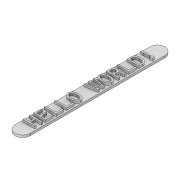
# Autodesk Inventor part: hello_world
Saved by Autodesk Inventor 2021 (Build 250183000, 183)
## iProperties
Created: 2021-09-21
Part Number: hello_world
Material: Generic
Document SubType Name: Modeling
Designer: Administrator
Density: 1 g/cm^3
Appearance: Default
Author: Administrator
Autodesk Inventor part; units mm, degrees
ref_plane "YZ Plane" through (0, 0, 0) normal (1, 0, 0) x (0, 1, 0)
ref_plane "XZ Plane" through (0, 0, 0) normal (0, 1, 0) x (-1, 0, 0)
ref_plane "XY Plane" through (0, 0, 0) normal (0, 0, 1) x (1, 0, 0)
sketch "Sketch1" plane through (0, 0, 0) normal (0, 1, 0) x (-1, 0, 0)
  line L0 (25, -250) -> (-25, -250)
  line L1 (-25, -250) -> (-25, 250)
  line L2 (-25, 250) -> (25, 250)
  line L3 (25, 250) -> (25, -250)
  line L4 (25, -250) -> (-25, 250) construction
  line L5 (-25, -250) -> (25, 250) construction
  point P0 (0, 0)
  dimension "d0" = 50
  dimension "d1" = 500
  constraints: 12 end point, 2 midpoint, 2 parallel, 1 horizontal, 1 perpendicular
  measures "d0" distance of L1.end L2.end
  measures "d1" distance of L0.end L1.end
extrude "Extrusion1" add sketch "Sketch1" along normal blind 7.5
fillet "Fillet1" radius 25 4 edges at (25, 3.75, 250) (-25, 3.75, 250) (25, 3.75, -250) (-25, 3.75, -250)
sketch "Sketch2" plane through (0, 7.5, 0) normal (0, 1, 0) x (1, 0, 0)
  line L0 (-21.1138, -208.405) -> (-21.1138, 208.4051) construction
  line L1 (-21.1138, 208.4051) -> (21.114, 208.4051) construction
  line L2 (21.114, 208.4051) -> (21.114, -208.405) construction
  line L3 (21.114, -208.405) -> (-21.1138, -208.405) construction
  line L4 (-25, 225) -> (-25, -225) projected
  arc A0 (-25, -225) -> (25, -225) centre (0, -225) ccw projected
  arc A1 (25, 225) -> (-25, 225) centre (0, 225) ccw projected
  line L5 (20.0001, -204.4219) -> (-19.9999, -204.4219)
  line L6 (-19.9999, -204.4219) -> (-19.9999, -199.0548)
  line L7 (-19.9999, -199.0548) -> (-3.6961, -199.0548)
  line L8 (-3.6961, -199.0548) -> (-3.6961, -183.0548)
  line L9 (-3.6961, -183.0548) -> (-19.9999, -183.0548)
  line L10 (-19.9999, -183.0548) -> (-19.9999, -177.7215)
  line L11 (-19.9999, -177.7215) -> (20.0001, -177.7215)
  line L12 (20.0001, -177.7215) -> (20.0001, -183.0548)
  line L13 (20.0001, -183.0548) -> (1.1984, -183.0548)
  line L14 (1.1984, -183.0548) -> (1.1984, -199.0548)
  line L15 (1.1984, -199.0548) -> (20.0001, -199.0548)
  line L16 (20.0001, -199.0548) -> (20.0001, -204.4219)
  line L17 (20.0001, -168.4388) -> (-19.9999, -168.4388)
  line L18 (-19.9999, -168.4388) -> (-19.9999, -143.5274)
  line L19 (-19.9999, -143.5274) -> (-15.1729, -143.5274)
  line L20 (-15.1729, -143.5274) -> (-15.1729, -163.1054)
  line L21 (-15.1729, -163.1054) -> (-3.156, -163.1054)
  line L22 (-3.156, -163.1054) -> (-3.156, -145.2489)
  line L23 (-3.156, -145.2489) -> (1.6372, -145.2489)
  line L24 (1.6372, -145.2489) -> (1.6372, -163.1054)
  line L25 (1.6372, -163.1054) -> (15.1731, -163.1054)
  line L26 (15.1731, -163.1054) -> (15.1731, -143.0885)
  line L27 (15.1731, -143.0885) -> (20.0001, -143.0885)
  line L28 (20.0001, -143.0885) -> (20.0001, -168.4388)
  line L29 (20.0001, -133.2658) -> (-19.9999, -133.2658)
  line L30 (-19.9999, -133.2658) -> (-19.9999, -127.9662)
  line L31 (-19.9999, -127.9662) -> (15.1731, -127.9662)
  line L32 (15.1731, -127.9662) -> (15.1731, -107.578)
  line L33 (15.1731, -107.578) -> (20.0001, -107.578)
  line L34 (20.0001, -107.578) -> (20.0001, -133.2658)
  line L35 (20.0001, -98.5316) -> (-19.9999, -98.5316)
  line L36 (-19.9999, -98.5316) -> (-19.9999, -93.232)
  line L37 (-19.9999, -93.232) -> (15.1731, -93.232)
  line L38 (15.1731, -93.232) -> (15.1731, -72.8438)
  line L39 (15.1731, -72.8438) -> (20.0001, -72.8438)
  line L40 (20.0001, -72.8438) -> (20.0001, -98.5316)
  spline S0 degree 2 poles (-0.0168, -66.9366) (-9.9746, -66.9366) (-21.1138, -59.0717) (-21.1138, -52.1181) knots 0 0 0 1 2 2 2
  spline S1 degree 2 poles (-21.1138, -52.1181) (-21.1138, -45.1982) (-9.8733, -37.2995) (-0.0168, -37.2995) knots 0 0 0 1 2 2 2
  spline S2 degree 2 poles (-0.0168, -37.2995) (9.8735, -37.2995) (21.114, -45.1982) (21.114, -52.1181) knots 0 0 0 1 2 2 2
  spline S3 degree 2 poles (21.114, -52.1181) (21.114, -59.0379) (9.8735, -66.9366) (-0.0168, -66.9366) knots 0 0 0 1 2 2 2
  spline S4 degree 2 poles (-0.0168, -61.4008) (7.6119, -61.4008) (16.287, -56.405) (16.287, -52.1181) knots 0 0 0 1 2 2 2
  spline S5 degree 2 poles (16.287, -52.1181) (16.287, -47.8312) (7.5781, -42.8354) (-0.0168, -42.8354) knots 0 0 0 1 2 2 2
  spline S6 degree 2 poles (-0.0168, -42.8354) (-7.6117, -42.8354) (-16.3206, -47.8312) (-16.3206, -52.1181) knots 0 0 0 1 2 2 2
  spline S7 degree 2 poles (-16.3206, -52.1181) (-16.3206, -56.405) (-7.6455, -61.4008) (-0.0168, -61.4008) knots 0 0 0 1 2 2 2
  line L41 (20.0001, 6.4473) -> (-20.0674, -0.4388)
  line L42 (-20.0674, -0.4388) -> (-20.0674, 4.287)
  line L43 (-20.0674, 4.287) -> (13.9916, 9.249)
  line L44 (13.9916, 9.249) -> (-20.0674, 14.7849)
  line L45 (-20.0674, 14.7849) -> (-20.0674, 19.8144)
  line L46 (-20.0674, 19.8144) -> (13.9916, 25.5191)
  line L47 (13.9916, 25.5191) -> (-20.0674, 30.4811)
  line L48 (-20.0674, 30.4811) -> (-20.0674, 35.1055)
  line L49 (-20.0674, 35.1055) -> (20.0001, 28.0507)
  line L50 (20.0001, 28.0507) -> (20.0001, 23.2237)
  line L51 (20.0001, 23.2237) -> (-14.7341, 17.249)
  line L52 (-14.7341, 17.249) -> (20.0001, 11.5444)
  line L53 (20.0001, 11.5444) -> (20.0001, 6.4473)
  spline S8 degree 2 poles (-0.0168, 37.2659) (-9.9746, 37.2659) (-21.1138, 45.1309) (-21.1138, 52.0845) knots 0 0 0 1 2 2 2
  spline S9 degree 2 poles (-21.1138, 52.0845) (-21.1138, 59.0043) (-9.8733, 66.903) (-0.0168, 66.903) knots 0 0 0 1 2 2 2
  spline S10 degree 2 poles (-0.0168, 66.903) (9.8735, 66.903) (21.114, 59.0043) (21.114, 52.0845) knots 0 0 0 1 2 2 2
  spline S11 degree 2 poles (21.114, 52.0845) (21.114, 45.1646) (9.8735, 37.2659) (-0.0168, 37.2659) knots 0 0 0 1 2 2 2
  spline S12 degree 2 poles (-0.0168, 42.8018) (7.6119, 42.8018) (16.287, 47.7975) (16.287, 52.0845) knots 0 0 0 1 2 2 2
  spline S13 degree 2 poles (16.287, 52.0845) (16.287, 56.3714) (7.5781, 61.3672) (-0.0168, 61.3672) knots 0 0 0 1 2 2 2
  spline S14 degree 2 poles (-0.0168, 61.3672) (-7.6117, 61.3672) (-16.3206, 56.3714) (-16.3206, 52.0845) knots 0 0 0 1 2 2 2
  spline S15 degree 2 poles (-16.3206, 52.0845) (-16.3206, 47.7975) (-7.6455, 42.8018) (-0.0168, 42.8018) knots 0 0 0 1 2 2 2
  line L54 (20.0001, 73.9579) -> (-19.9999, 73.9579)
  line L55 (-19.9999, 73.9579) -> (-19.9999, 87.325)
  spline S16 degree 2 poles (-19.9999, 87.325) (-19.9999, 93.2321) (-14.1603, 99.4431) (-8.5906, 99.4431) knots 0 0 0 1 2 2 2
  spline S17 degree 2 poles (-8.5906, 99.4431) (-5.2826, 99.4431) (-0.7257, 96.7764) (0.4895, 94.1773) knots 0 0 0 1 2 2 2
  spline S18 degree 2 poles (0.4895, 94.1773) (1.1646, 96.3376) (4.1013, 98.2617) (7.8144, 98.5317) knots 0 0 0 1 2 2 2
  line L56 (7.8144, 98.5317) -> (14.3292, 98.9368)
  spline S19 degree 2 poles (14.3292, 98.9368) (16.422, 99.0718) (18.3798, 99.8819) (18.8862, 100.7258) knots 0 0 0 1 2 2 2
  line L57 (18.8862, 100.7258) -> (20.0001, 100.7258)
  line L58 (20.0001, 100.7258) -> (20.0001, 94.6499)
  spline S20 degree 2 poles (20.0001, 94.6499) (19.3587, 94.2785) (16.7596, 93.7722) (14.5655, 93.6372) knots 0 0 0 1 2 2 2
  line L59 (14.5655, 93.6372) -> (9.4009, 93.3334)
  spline S21 degree 2 poles (9.4009, 93.3334) (5.4853, 93.1309) (3.1224, 90.3629) (3.1224, 84.7933) knots 0 0 0 1 2 2 2
  line L60 (3.1224, 84.7933) -> (3.1224, 79.2912)
  line L61 (3.1224, 79.2912) -> (20.0001, 79.2912)
  line L62 (20.0001, 79.2912) -> (20.0001, 73.9579)
  line L63 (-15.1054, 85.8397) -> (-15.1054, 79.2912)
  line L64 (-15.1054, 79.2912) -> (-1.7721, 79.2912)
  line L65 (-1.7721, 79.2912) -> (-1.7721, 85.4684)
  spline S22 degree 2 poles (-1.7721, 85.4684) (-1.7721, 90.1942) (-4.8776, 93.9072) (-8.4894, 93.9072) knots 0 0 0 1 2 2 2
  spline S23 degree 2 poles (-8.4894, 93.9072) (-12.0337, 93.9072) (-15.1054, 90.2279) (-15.1054, 85.8397) knots 0 0 0 1 2 2 2
  line L66 (20.0001, 109.8735) -> (-19.9999, 109.8735)
  line L67 (-19.9999, 109.8735) -> (-19.9999, 115.1731)
  line L68 (-19.9999, 115.1731) -> (15.1731, 115.1731)
  line L69 (15.1731, 115.1731) -> (15.1731, 135.5612)
  line L70 (15.1731, 135.5612) -> (20.0001, 135.5612)
  line L71 (20.0001, 135.5612) -> (20.0001, 109.8735)
  spline S24 degree 2 poles (-19.9999, 156.2532) (-19.9999, 163.7469) (-10.0759, 171.1393) (-0.0168, 171.1393) knots 0 0 0 1 2 2 2
  spline S25 degree 2 poles (-0.0168, 171.1393) (9.5697, 171.1393) (20.0001, 163.3756) (20.0001, 156.2532) knots 0 0 0 1 2 2 2
  line L72 (20.0001, 156.2532) -> (20.0001, 142.9199)
  line L73 (20.0001, 142.9199) -> (-19.9999, 142.9199)
  line L74 (-19.9999, 142.9199) -> (-19.9999, 156.2532)
  line L75 (-15.2067, 155.8482) -> (-15.2067, 148.287)
  line L76 (-15.2067, 148.287) -> (15.2068, 148.287)
  line L77 (15.2068, 148.287) -> (15.2068, 155.8482)
  spline S26 degree 2 poles (15.2068, 155.8482) (15.2068, 160.8102) (7.7132, 165.6034) (-0.0168, 165.6034) knots 0 0 0 1 2 2 2
  spline S27 degree 2 poles (-0.0168, 165.6034) (-8.0843, 165.6034) (-15.2067, 161.0465) (-15.2067, 155.8482) knots 0 0 0 1 2 2 2
  line L78 (8.0845, 189.5697) -> (-8.3206, 188.1857)
  line L79 (-8.3206, 188.1857) -> (-20.0674, 188.1857)
  line L80 (-20.0674, 188.1857) -> (-20.0674, 193.8566)
  line L81 (-20.0674, 193.8566) -> (-8.3206, 193.8566)
  line L82 (-8.3206, 193.8566) -> (8.0845, 192.5401)
  line L83 (8.0845, 192.5401) -> (8.0845, 189.5697)
  line L84 (20.0001, 186.9705) -> (11.4262, 186.9705)
  line L85 (11.4262, 186.9705) -> (11.4262, 195.0043)
  line L86 (11.4262, 195.0043) -> (20.0001, 195.0043)
  line L87 (20.0001, 195.0043) -> (20.0001, 186.9705)
  dimension "d6" = 0
  dimension "d8" = 21.114
  dimension "d9" = 433.405
  constraints: 2 other
  measures "d6" angle of L4 L0
  measures "d8" distance from line of A0.centre L2
  measures "d9" distance from line of A1.centre L3
extrude "Extrusion2" add sketch "Sketch2" along normal blind 7.5
body "Solid1"
